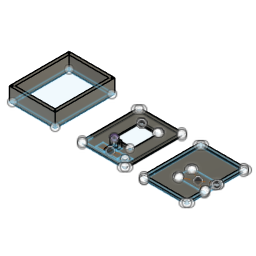
HACZYK_OBUDOWA v1 (Autodesk Fusion 360 design; units mm, degrees)
Autodesk Fusion 360 part; units mm, degrees
sketch "Szkic1" plane through (0, 0, 0) normal (0, 0, 1) x (1, 0, 0)
  line L0 (0, 0) -> (34.05, 0)
  line L1 (34.05, 0) -> (34.05, 46)
  line L2 (34.05, 46) -> (0, 46)
  line L3 (0, 46) -> (0, 0)
  line L4 (54.05, -20) -> (54.05, 66)
  line L5 (54.05, 66) -> (-20, 66)
  line L6 (-20, 66) -> (-20, -20)
  line L7 (0, 46) -> (34.05, 46)
  line L8 (34.05, 46) -> (34.05, 50.85)
  line L9 (34.05, 50.85) -> (0, 50.85)
  line L10 (0, 50.85) -> (0, 46)
  line L11 (0, 0) -> (34.05, 0)
  line L12 (34.05, 0) -> (34.05, -4.85)
  line L13 (34.05, -4.85) -> (0, -4.85)
  line L14 (0, -4.85) -> (0, 0)
  line L15 (34.05, 50.85) -> (33.05, 50.85)
  line L16 (34.05, 49.85) -> (34.05, 50.85)
  line L17 (33.05, 49.85) -> (32.7581, 49.85)
  circle A0 centre (31.55, 48.35) radius 1.55
  line L18 (0, 50.85) -> (1, 50.85)
  line L19 (0, 49.85) -> (0, 50.85)
  line L20 (2.5, 49.85) -> (2.5, 48.35)
  circle A1 centre (2.5, 48.35) radius 1.55
  circle A2 centre (2.5, -2.65) radius 1.55
  circle A3 centre (31.55, -2.65) radius 1.55
  line L21 (-20, -20) -> (-20, -34)
  line L22 (54.05, -20) -> (54.05, -34)
  line L23 (54.05, -34) -> (-20, -34)
  line L24 (37.025, -30.925) -> (-2.975, -30.925)
  line L25 (-2.975, -30.925) -> (-2.975, -17.925)
  line L26 (-2.975, -17.925) -> (37.025, -17.925)
  line L27 (37.025, -17.925) -> (37.025, -30.925)
  line L28 (37.025, -30.925) -> (-2.975, -17.925) construction
  line L29 (-2.975, -30.925) -> (37.025, -17.925) construction
  line L30 (19.975, -30.925) -> (14.075, -30.925)
  line L31 (14.075, -30.925) -> (14.075, -17.925)
  line L32 (14.075, -17.925) -> (19.975, -17.925)
  line L33 (19.975, -17.925) -> (19.975, -30.925)
  line L34 (19.975, -30.925) -> (14.075, -17.925) construction
  line L35 (14.075, -30.925) -> (19.975, -17.925) construction
  line L36 (14.075, -17.925) -> (10.075, -17.925)
  line L37 (10.075, -17.925) -> (10.075, -9.925)
  line L38 (10.075, -9.925) -> (14.075, -9.925)
  line L39 (14.075, -9.925) -> (14.075, -17.925)
  line L40 (19.975, -17.925) -> (23.975, -17.925)
  line L41 (23.975, -17.925) -> (23.975, -9.925)
  line L42 (23.975, -9.925) -> (19.975, -9.925)
  line L43 (19.975, -9.925) -> (19.975, -17.925)
  line L44 (14.075, -17.925) -> (12.075, -17.925)
  line L45 (12.075, -17.925) -> (12.075, -30.925)
  line L46 (12.075, -30.925) -> (14.075, -30.925)
  line L47 (14.075, -30.925) -> (14.075, -17.925)
  line L48 (19.975, -17.925) -> (21.975, -17.925)
  line L49 (21.975, -17.925) -> (21.975, -30.925)
  line L50 (21.975, -30.925) -> (19.975, -30.925)
  line L51 (19.975, -30.925) -> (19.975, -17.925)
  line L52 (37.025, -30.925) -> (51.025, -30.925)
  line L53 (51.025, -30.925) -> (51.025, -16.925)
  line L54 (51.025, -16.925) -> (37.025, -16.925)
  line L55 (37.025, -16.925) -> (37.025, -30.925)
  circle A4 centre (44.025, -23.925) radius 3.35
  line L56 (-25.5, -20) -> (-25.5, -39.5)
  line L57 (59.55, -39.5) -> (-25.5, -39.5)
  line L58 (59.55, -20) -> (59.55, -39.5)
  line L59 (59.55, -20) -> (59.55, 71.5)
  line L60 (59.55, 71.5) -> (-25.5, 71.5)
  line L61 (-25.5, 71.5) -> (-25.5, -20)
  line L62 (-25.5, 66) -> (-25.5, 71.5)
  line L63 (-25.5, 71.5) -> (-20, 71.5)
  circle A5 centre (-22.75, 68.75) radius 1.55
  line L64 (59.55, 66) -> (59.55, 71.5)
  line L65 (59.55, 71.5) -> (54.05, 71.5)
  circle A6 centre (56.8, 68.75) radius 1.55
  line L66 (59.55, -34) -> (59.55, -39.5)
  line L67 (59.55, -39.5) -> (54.05, -39.5)
  line L68 (-25.5, -34) -> (-25.5, -39.5)
  line L69 (-25.5, -39.5) -> (-20, -39.5)
  circle A7 centre (56.8, -36.75) radius 1.55
  circle A8 centre (-22.75, -36.75) radius 1.55
  circle A9 centre (171.8, 68.75) radius 1.55
  line L70 (174.55, 71.5) -> (169.05, 71.5)
  line L71 (169.05, -34) -> (95, -34)
  line L72 (95, 66) -> (95, -20)
  line L73 (169.05, 66) -> (95, 66)
  line L74 (169.05, -20) -> (169.05, -34)
  circle A10 centre (171.8, -36.75) radius 1.55
  line L75 (95, -20) -> (95, -34)
  line L76 (174.55, -39.5) -> (169.05, -39.5)
  line L77 (89.5, 66) -> (89.5, 71.5)
  line L78 (89.5, 71.5) -> (95, 71.5)
  circle A11 centre (92.25, 68.75) radius 1.55
  line L79 (174.55, -34) -> (174.55, -39.5)
  line L80 (89.5, -34) -> (89.5, -39.5)
  line L81 (89.5, -39.5) -> (95, -39.5)
  line L82 (89.5, -20) -> (89.5, -39.5)
  line L83 (174.55, -39.5) -> (89.5, -39.5)
  line L84 (174.55, -20) -> (174.55, -39.5)
  line L85 (174.55, -20) -> (174.55, 71.5)
  line L86 (174.55, 71.5) -> (89.5, 71.5)
  line L87 (89.5, 71.5) -> (89.5, -20)
  circle A12 centre (92.25, -36.75) radius 1.55
  line L88 (172.5995, 23.2495) -> (120.8995, 23.2495)
  line L89 (120.8995, 23.2495) -> (120.8995, -5.2005)
  line L90 (120.8995, -5.2005) -> (172.5995, -5.2005)
  line L91 (172.5995, -5.2005) -> (120.8995, 23.2495) construction
  line L92 (172.5995, 23.2495) -> (120.8995, -5.2005) construction
  line L93 (172.5995, -5.2005) -> (172.5995, -4.1005)
  line L94 (171.4995, -5.2005) -> (172.5995, -5.2005)
  line L95 (172.5995, 23.2495) -> (172.5995, 22.1495)
  line L96 (171.4995, 23.2495) -> (172.5995, 23.2495)
  line L97 (120.8995, -5.2005) -> (120.8995, -4.1005)
  line L98 (121.9995, -5.2005) -> (120.8995, -5.2005)
  line L99 (120.8995, 23.2495) -> (120.8995, 22.1495)
  line L100 (121.9995, 23.2495) -> (120.8995, 23.2495)
  line L101 (120.8995, -5.2005) -> (120.8995, -1.1005)
  line L102 (124.9995, -5.2005) -> (120.8995, -5.2005)
  circle A13 centre (123.4995, -2.6005) radius 1.5
  line L103 (120.8995, 23.2495) -> (120.8995, 19.1495)
  line L104 (124.9995, 23.2495) -> (120.8995, 23.2495)
  circle A14 centre (123.4995, 20.6495) radius 1.5
  line L105 (172.5995, 23.2495) -> (172.5995, 19.1495)
  line L106 (168.4995, 23.2495) -> (172.5995, 23.2495)
  line L107 (172.5995, -5.2005) -> (172.5995, -1.1005)
  line L108 (168.4995, -5.2005) -> (172.5995, -5.2005)
  circle A15 centre (169.9995, -2.6005) radius 1.5
  circle A16 centre (169.9995, 20.6495) radius 1.5
  line L109 (169.05, 23.2495) -> (169.05, 66)
  line L110 (170.6006, 22.1495) -> (169.9995, 22.1495)
  line L111 (169.05, -20) -> (169.05, -5.2005)
  line L112 (172.5995, 19.1495) -> (172.5995, 18.6495)
  line L113 (168.4995, 23.2495) -> (168.4995, -5.2005)
  line L114 (172.5995, -1.1005) -> (172.5995, -0.6)
  line L115 (168.4995, 23.2495) -> (172.5995, 23.2495)
  line L116 (172.5995, 23.2495) -> (172.5995, 18.6495)
  line L117 (168.4995, 17.2495) -> (168.4995, 23.2495)
  line L118 (172.5995, -5.2005) -> (168.4995, -5.2005)
  line L119 (168.4995, -5.2005) -> (168.4995, 0.7995)
  line L120 (172.5995, -0.6) -> (172.5995, -5.2005)
  line L121 (172.5995, -5.2005) -> (172.5995, -0.6)
  line L122 (172.5995, 18.6495) -> (172.5995, 23.2495)
  line L123 (169.9995, -0.6005) -> (172.5995, -0.6)
  line L124 (169.9995, -0.6005) -> (168.4995, -0.6002)
  line L125 (169.9995, 20.6495) -> (169.9995, 18.6495)
  line L126 (168.4995, 18.6642) -> (172.5995, 18.6495)
  line L127 (172.5995, 23.2495) -> (174.55, 23.2495)
  line L128 (172.5995, -5.2005) -> (174.55, -5.2005)
  line L129 (-75.95, 66) -> (-150, 66)
  line L130 (-70.45, 71.5) -> (-155.5, 71.5)
  line L131 (-155.5, 71.5) -> (-155.5, -20)
  line L132 (-150, 66) -> (-150, -20)
  circle A17 centre (-152.75, 68.75) radius 1.55
  circle A18 centre (-73.2, 68.75) radius 1.55
  line L133 (-75.95, -20) -> (-75.95, 66)
  line L134 (-70.45, -20) -> (-70.45, 71.5)
  line L135 (-150, -20) -> (-150, -34)
  line L136 (-155.5, -20) -> (-155.5, -39.5)
  line L137 (-75.95, -34) -> (-150, -34)
  line L138 (-70.45, -39.5) -> (-155.5, -39.5)
  circle A19 centre (-152.75, -36.75) radius 1.55
  line L139 (-70.45, -20) -> (-70.45, -39.5)
  line L140 (-75.95, -20) -> (-75.95, -34)
  circle A20 centre (-73.2, -36.75) radius 1.55
  point P0 (17.025, -24.425)
  point P1 (17.025, -24.425)
  point P2 (95, -39.5)
  point P3 (174.55, 66)
  point P4 (146.7495, 9.0245)
  dimension "d1" = 34.05
  dimension "d2" = 46
  dimension "d5" = 4.85
  dimension "d6" = 4.85
  dimension "d7" = 1
  dimension "d11" = 3.1
  dimension "d14" = 1.5
  dimension "d15" = 3.1
  dimension "d16" = 3.1
  dimension "d17" = 3.1
  dimension "d22" = 13
  dimension "d23" = 5.9
  dimension "d24" = 4
  dimension "d25" = 8
  dimension "d26" = 4
  dimension "d27" = 8
  dimension "d28" = 2
  dimension "d29" = 13
  dimension "d30" = 13
  dimension "d31" = 14
  dimension "d32" = 14
  dimension "d33" = 6.7
  dimension "d38" = 5.5
  dimension "d39" = 3.1
  dimension "d40" = 3.1
  dimension "d41" = 3.1
  dimension "d42" = 3.1
  dimension "d68" = 3.1
  dimension "d69" = 3.1
  dimension "d70" = 3.1
  dimension "d71" = 3.1
  dimension "d72" = 28.45
  dimension "d73" = 51.7
  dimension "d74" = 1.1
  dimension "d75" = 1.1
  dimension "d76" = 1.1
  dimension "d77" = 1.1
  dimension "d78" = 1.1
  dimension "d79" = 1.1
  dimension "d80" = 1.1
  dimension "d81" = 1.1
  dimension "d82" = 4.1
  dimension "d83" = 4.1
  dimension "d84" = 4.1
  dimension "d85" = 4.1
  dimension "d86" = 4.1
  dimension "d87" = 4.1
  dimension "d90" = 0.5
  dimension "d91" = 6
  dimension "d101" = 2
  dimension "d102" = 2
  dimension "d107" = 5.5
  dimension "d108" = 3.1
  dimension "d109" = 3.1
  dimension "d110" = 3.1
  dimension "d111" = 3.1
  constraint horizontal L0
  constraint vertical L1
  constraint horizontal L2
  constraint vertical L3
  constraint coincident L0.start L3.end
  constraint horizontal L7
  constraint vertical L8
  constraint horizontal L9
  constraint vertical L10
  constraint horizontal L11
  constraint vertical L12
  constraint horizontal L13
  constraint vertical L14
  constraint horizontal L15
  constraint vertical L16
  constraint horizontal L18
  constraint vertical L19
  constraint coincident L20.end A1.centre
  constraint parallel L4 L22
  constraint perpendicular L21 L23
  constraint horizontal L24
  constraint perpendicular L24 L25
  constraint parallel L24 L26
  constraint parallel L25 L27
  constraint coincident L28 P1
  constraint coincident L29 P1
  constraint horizontal L30
  constraint perpendicular L30 L31
  constraint parallel L30 L32
  constraint parallel L31 L33
  constraint coincident L34 P1
  constraint coincident L35 P1
  constraint coincident P1 P0
  constraint horizontal L36
  constraint vertical L37
  constraint horizontal L38
  constraint vertical L39
  constraint horizontal L40
  constraint vertical L41
  constraint horizontal L42
  constraint vertical L43
  constraint horizontal L44
  constraint vertical L45
  constraint horizontal L46
  constraint vertical L47
  constraint horizontal L48
  constraint vertical L49
  constraint horizontal L50
  constraint vertical L51
  constraint horizontal L52
  constraint vertical L53
  constraint horizontal L54
  constraint vertical L55
  constraint vertical L62
  constraint horizontal L63
  constraint vertical L64
  constraint horizontal L65
  constraint vertical L66
  constraint horizontal L67
  constraint vertical L68
  constraint horizontal L69
  constraint parallel L74 L111
  constraint perpendicular L71 L75
  constraint vertical L77
  constraint horizontal L78
  constraint horizontal L70
  constraint vertical L79
  constraint horizontal L76
  constraint vertical L80
  constraint horizontal L81
  constraint perpendicular L88 L121
  constraint parallel L89 L121
  constraint parallel L88 L90
  constraint coincident L91 P4
  constraint coincident L92 P4
  constraint coincident L88 L109.start
  constraint collinear L109 L111
  constraint coincident L92 L110.start
  constraint coincident A16 L110.end
  constraint coincident L90 L111.end
  constraint parallel L112 L121
  constraint perpendicular L90 L113
  constraint parallel L114 L121
  constraint horizontal L115
  constraint vertical L116
  constraint vertical L117
  constraint horizontal L118
  constraint vertical L119
  constraint vertical L120
  constraint collinear L121 L122
  constraint coincident L113 L124.end
  constraint coincident A16.centre L125.start
  constraint vertical L125
  constraint coincident L113 L126.start
  constraint coincident L85 L127.end
  constraint perpendicular L85 L127
  constraint coincident L85 L128.end
  constraint perpendicular L85 L128
  constraint parallel L133 L140
  constraint perpendicular L135 L137
  measures "d1" distance of L0.start L0.end
  measures "d2" distance of L0.start L2.end
  measures "d5" distance of L2.end L9.end
  measures "d6" distance of L0.start L13.end
  measures "d7" distance of L8.end L15.end
  measures "d11" diameter of A0
  measures "d14" distance of L20.start L20.end
  measures "d15" diameter of A1
  measures "d16" diameter of A2
  measures "d17" diameter of A3
  measures "d22" distance of L24.end L25.end
  measures "d23" distance of L31.end L32.end
  measures "d24" distance of L31.end L36.end
  measures "d25" distance of L31.end L38.end
  measures "d26" distance of L32.end L40.end
  measures "d27" distance of L32.end L42.end
  measures "d28" distance of L31.end L44.end
  measures "d29" distance of L31.end L30.end
  measures "d30" distance of L32.end L30.start
  measures "d31" distance of L24.start L52.end
  measures "d32" distance of L24.start L54.end
  measures "d33" diameter of A4
  measures "d39" diameter of A5
  measures "d40" diameter of A6
  measures "d41" diameter of A7
  measures "d42" diameter of A8
  measures "d68" diameter of A11
  measures "d69" diameter of A9
  measures "d70" diameter of A10
  measures "d71" diameter of A12
  measures "d72" distance of L88.end L89.end
  measures "d73" distance of L88.start L88.end
  measures "d74" distance of L90.end L93.end
  measures "d75" distance of L90.end L94.start
  measures "d76" distance of L88.start L95.end
  measures "d77" distance of L88.start L96.start
  measures "d78" distance of L89.end L97.end
  measures "d79" distance of L89.end L98.start
  measures "d80" distance of L88.end L99.end
  measures "d81" distance of L88.end L100.start
  measures "d82" distance of L89.end L101.end
  measures "d83" distance of L89.end L102.start
  measures "d84" distance of L88.end L103.end
  measures "d85" distance of L88.end L104.start
  measures "d86" distance of L88.start L105.end
  measures "d87" distance of L88.start L106.start
  measures "d90" distance of L105.end L112.end
  measures "d91" distance of L106.start L117.start
  measures "d101" distance of A15.centre L123.start
  measures "d102" distance of A16.centre L125.end
  measures "d108" diameter of A17
  measures "d109" diameter of A18
  measures "d110" diameter of A20
  measures "d111" diameter of A19
extrude "Wyciągnięcie proste1" add sketch "Szkic1" along normal blind 1 contours L4 L5 L6 L21 L22 L23 | L24 L26 L27 L40 L49 L55 | L27 L52 L53 L54 L55 | L24 L25 L26 L36 L45 makes body 1
extrude "Wyciągnięcie proste2" add sketch "Szkic1" along normal blind 1 contours L0 L11 L12 L13 L14 | L2 L7 L8 L9 L10 L15 L16 L18 L19 bodies 1
extrude "Wyciągnięcie proste3" add sketch "Szkic1" along normal blind 1 contours L56 L57 L58 L59 L60 L61 L62 L63 L64 L65 L66 L67 L68 L69 bodies 1
extrude "Wyciągnięcie proste4" add sketch "Szkic1" along normal blind 5 separate body contours L24 L26 L33 L40 L48 L49 L50 L51 | L24 L26 L31 L36 L44 L45 L46 L47 makes body 2 at (21.975, -22.2583, 1.6667) makes body 3 at (12.075, -22.2583, 1.6667)
extrude "Wyciągnięcie proste5" add sketch "Szkic1" along normal blind 15 contours L26 L40 L41 L42 L43 L48 | L26 L36 L37 L38 L39 L44 bodies 1 2 3
extrude "Wyciągnięcie proste6" add sketch "Szkic1" along normal blind 1 separate body contours L71 L72 L73 L74 L75 L88 L89 L90 L97 L98 L99 L100 L101 L102 L103 L104 L106 L108 L109 L111 L115 L118 makes body 4
extrude "Wyciągnięcie proste7" add sketch "Szkic1" along normal blind 1 contours L88 L95 L96 L105 L106 A16 L112 L113 L115 L116 L117 L122 L125 L126 | L90 L93 L94 L107 L108 L113 L114 L118 L119 L120 L121 L123 L124 | L88 L89 L90 L97 L98 L99 L100 L101 L102 L103 L104 L113 L117 L119 | A16 L113 L117 L125 L126 bodies 4
extrude "Wyciągnięcie proste8" add sketch "Szkic1" along normal blind 3 contours L70 L71 L72 L73 L74 L75 L76 L77 L78 L79 L80 L81 L82 L83 L84 L85 L86 L87 L88 L90 L94 L96 L106 L108 L109 L111 L115 L118 L127 L128 bodies 4
extrude "Wyciągnięcie proste9" add sketch "Szkic1" along normal blind 26 separate body contours L130 L131 L134 L136 L138 L139 makes body 5
sketch "Szkic3" plane through (0, 0, 0) normal (1, 0, 0) x (0, 1, 0)
  line L0 (-18, 15) -> (-10, 15)
  line L1 (-10, 15) -> (-10, 7)
  line L2 (-10, 7) -> (-18, 7)
  line L3 (-18, 7) -> (-18, 15)
  circle A0 centre (-14, 11) radius 4
  circle A1 centre (-14, 11) radius 1.5
  dimension "d114" = 8
  dimension "d115" = 8
  dimension "d125" = 3
  constraint horizontal L0
  constraint vertical L1
  constraint horizontal L2
  constraint vertical L3
  constraint tangent L3 A0
  constraint tangent L0 A0
  constraint tangent L1 A0
  constraint concentric A0 A1
  measures "d114" distance of L0.start L0.end
  measures "d115" distance of L0.start L2.end
  measures "d125" diameter of A1
sketch "Szkic4" plane through (0, 0, 0) normal (1, 0, 0) x (0, 1, 0)
  line L0 (-31, 5) -> (-18, 5)
  line L1 (-18, 5) -> (-18, 3)
  line L2 (-18, 3) -> (-31, 3)
  line L3 (-31, 3) -> (-31, 5)
  line L4 (-31, 5) -> (-29, 5)
  line L5 (-29, 5) -> (-29, 3)
  line L6 (-29, 3) -> (-31, 3)
  line L7 (-31, 3) -> (-31, 5)
  line L8 (-18, 5) -> (-20.2, 5)
  line L9 (-20.2, 5) -> (-20.2, 3)
  line L10 (-20.2, 3) -> (-18, 3)
  line L11 (-18, 3) -> (-18, 5)
  line L12 (-29, 5) -> (-27, 5)
  line L13 (-27, 5) -> (-27, 3)
  line L14 (-27, 3) -> (-29, 3)
  line L15 (-29, 3) -> (-29, 5)
  line L16 (-20.2, 5) -> (-22.2, 5)
  line L17 (-22.2, 5) -> (-22.2, 3)
  line L18 (-22.2, 3) -> (-20.2, 3)
  line L19 (-20.2, 3) -> (-20.2, 5)
  circle A0 centre (-28, 4) radius 1
  circle A1 centre (-21.2, 4) radius 1
  circle A2 centre (-28, 4) radius 0.75
  circle A3 centre (-21.2, 4) radius 0.75
  dimension "d117" = 2
  dimension "d118" = 2.2
  dimension "d119" = 2
  dimension "d120" = 2
  dimension "d121" = 2
  dimension "d122" = 2
  dimension "d123" = 1.5
  dimension "d124" = 1.5
  constraint horizontal L0
  constraint vertical L1
  constraint horizontal L2
  constraint vertical L3
  constraint horizontal L4
  constraint vertical L5
  constraint horizontal L6
  constraint vertical L7
  constraint horizontal L8
  constraint vertical L9
  constraint horizontal L10
  constraint vertical L11
  constraint horizontal L12
  constraint vertical L13
  constraint horizontal L14
  constraint vertical L15
  constraint horizontal L16
  constraint vertical L17
  constraint horizontal L18
  constraint vertical L19
  constraint tangent L5 A0
  constraint tangent L0 A0
  constraint tangent L13 A0
  constraint tangent L17 A1
  constraint tangent L16 A1
  constraint tangent L9 A1
  constraint concentric A0 A2
  constraint concentric A1 A3
  measures "d117" distance of L0.start L4.end
  measures "d118" distance of L0.end L8.end
  measures "d119" distance of L0.end L1.end
  measures "d120" distance of L4.end L12.end
  measures "d121" distance of L8.end L16.end
  measures "d122" distance of L8.end L9.end
  measures "d123" diameter of A2
  measures "d124" diameter of A3
extrude "Wyciągnięcie proste10" cut sketch "Szkic3" sketch "Szkic4" along normal blind 27 contours A1 of sketch 2 contours A2 | A3 bodies 1
chamfer "Fazowanie1" distance 0.5 angle 45 4 edges at (0, 23, 1) (17.025, 46, 1) (34.05, 23, 1) (17.025, 0, 1) on bodies 1
fillet "Zaokrąglenie1" radius 2.5 4 edges at (21.975, -9.925, 15) (21.975, -17.925, 15) (12.075, -17.925, 15) (12.075, -9.925, 15) on bodies 1
fillet "Zaokrąglenie2" radius 2.5 2 edges at (20.975, -30.925, 5) (13.075, -30.925, 5) on bodies 1
